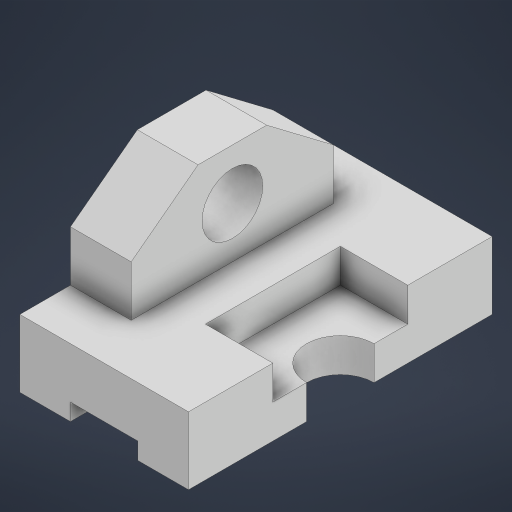
# Autodesk Inventor part: Część13
Saved by Autodesk Inventor 2023 (Build 270158000, 158)
## iProperties
Created: 2023-05-07
Part Number: Część13
Material: Ogólny
Document SubType Name: Modeling
Designer: Adam
Density: 1 g/cm^3
Appearance: Domyślna
Author: Adam
Autodesk Inventor part; units mm, degrees
ref_plane "YZ Plane" through (0, 0, 0) normal (1, 0, 0) x (0, 1, 0)
ref_plane "XZ Plane" through (0, 0, 0) normal (0, 1, 0) x (-1, 0, 0)
ref_plane "XY Plane" through (0, 0, 0) normal (0, 0, 1) x (1, 0, 0)
sketch "Szkic1" plane through (0, 0, 0) normal (0, 1, 0) x (-1, 0, 0)
  line L0 (0, 0) -> (-50, 0)
  line L1 (-50, 0) -> (-50, -90)
  line L2 (-50, -90) -> (0, -90)
  line L3 (0, -90) -> (0, 0)
  dimension "d0" = 50
  dimension "d1" = 90
  constraints: 8 end point, 2 parallel, 1 coincident, 1 horizontal, 1 perpendicular
  measures "d0" distance of L2.end L1.end
  measures "d1" distance of L1.end L0.end
extrude "Wyciągnięcie proste1" add sketch "Szkic1" along normal blind 20
sketch "Szkic2" plane through (0, 20, 0) normal (0, 1, 0) x (1, 0, 0)
  line L0 (50, 0) -> (50, 90) projected
  line L1 (50, 65) -> (30, 65)
  line L2 (30, 65) -> (30, 25)
  line L3 (30, 25) -> (50, 25)
  line L4 (50, 25) -> (50, 65)
  line L5 (50, 90) -> (0, 90) projected
  point P0 (0, 0)
  dimension "d4" = 20
  dimension "d5" = 40
  dimension "d6" = 25
  constraints: 8 end point, 2 parallel, 1 horizontal, 1 perpendicular, 1 point on line
  measures "d4" distance of L3.end L2.end
  measures "d5" distance of L2.end L1.end
  measures "d6" distance between parallel lines of L1 L5
extrude "Wyciągnięcie proste2" cut sketch "Szkic2" against normal blind 10
sketch "Szkic3" plane through (0, 10, 0) normal (0, 1, 0) x (1, 0, 0)
  line L0 (50, 65) -> (50, 25) projected
  circle A0 centre (50, 45) radius 10
  point P0 (0, 0)
  point P1 (50, 35)
  point P2 (50, 55)
  dimension "d9" = 20
  constraints: 1 centre point, 1 midpoint
  measures "d9" diameter of A0
extrude "Wyciągnięcie proste3" cut sketch "Szkic3" against normal through all contours L0 A0 picked at (46.1942, 47.495)
sketch "Szkic4" plane through (0, 0, 0) normal (0, -1, 0) x (1, 0, 0)
  line L0 (0, 0) -> (50, 0) projected
  line L1 (50, -90) -> (0, -90) projected
  line L2 (15, 0) -> (35, 0)
  line L3 (35, 0) -> (35, -90)
  line L4 (35, -90) -> (15, -90)
  line L5 (15, -90) -> (15, 0)
  line L6 (0, -90) -> (0, 0) projected
  dimension "d12" = 20
  dimension "d13" = 15
  constraints: 8 end point, 2 parallel, 2 point on line, 1 horizontal, 1 perpendicular
  measures "d12" distance of L3.end L4.end
  measures "d13" distance between parallel lines of L5 L6
extrude "Wyciągnięcie proste4" cut sketch "Szkic4" against normal blind 5 contours L0 L3 L1 L5
sketch "Szkic5" plane through (0, 0, 0) normal (1, 0, 0) x (0, 1, 0)
  line L0 (20, -65) -> (20, -90) projected
  line L1 (20, -75) -> (35, -75)
  line L2 (35, -75) -> (50, -55.1735)
  line L3 (50, -55.1735) -> (50, -45.1735)
  line L4 (20, -25) -> (20, -65) projected
  line L5 (20, -15) -> (35, -15)
  line L6 (35, -15) -> (50, -34.8265)
  line L7 (50, -34.8265) -> (50, -44.8265)
  line L8 (20, -75) -> (20, -15)
  line L9 (20, -90) -> (20, 0) projected
  line L10 (50, -55.1735) -> (50, -34.8265)
  point P0 (0, 0)
  dimension "d16" = 15
  dimension "d17" = 10
  dimension "d18" = 15
  constraints: 16 end point, 1 collinear, 1 horizontal, 1 perpendicular, 1 point on line, 1 vertical
  measures "d16" distance of L1.start L1.end
  measures "d17" distance of L2.end L3.end
  measures "d18" distance from line of L1.end L3
extrude "Wyciągnięcie proste5" add sketch "Szkic5" along normal blind 18
sketch "Szkic6" plane through (18, 0, 0) normal (1, 0, 0) x (0, 0, -1)
  line L0 (25, 20) -> (65, 20) projected
  line L1 (15, 35) -> (15, 20) projected
  point P0 (0, 0)
  point P1 (45, 35)
  point P2 (45, 20)
  point P3 (15, 27.5)
  dimension "d21" = 15
  dimension "d22" = 30
  constraints: 2 midpoint
  measures "d21" distance of point (45, 20) point (45, 35)
  measures "d22" horizontal distance of point (15, 27.5) point (45, 35)
hole "Otwór1" at (18, 35, -45) direction (-1, 0, 0) diameter 18 end through all
